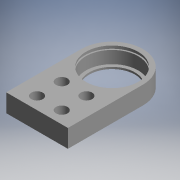
# Autodesk Inventor part: SBGSMA6006ZZ-40_h
Saved by Autodesk Inventor 2017.3 (Build 213256000, 256)
## iProperties
Part Number: SBGSMA6006ZZ-40_h
Material: Generic
Catalog Web Link: www.cadenas.de
Description: BGSMA, BGSMAB, SBGSMA_housing-Bearing with Housings - Front Installation Type
Vendor: MISUMI
Document SubType Name: Modeling
Designer: partserver
Manufacturer: MISUMI
Mass: 75.9528 g
Surface Area: 218.968 cm^2
Volume: 75.9528 cm^3
Density: 1 g/cm^3
Appearance: PSOLRGB-192-192-192
Category: PARTsolutions
Company: MISUMI
Title: SBGSMA6006ZZ-40
Author: Cadenas PARTsolutions
Comments: Bearing with Housings - Front Installation Type
PSOL_IDENT_0: {$CADENAS_DATA\23d-libs\misumi\metric\12_bearing_holders\bgsma\bgsma_housing.prj},219 {VTYP=3D},{NB=
PSOL_IDENT_1: SBGSMA6006ZZ-40_h},{LINA=SBGSMA6006ZZ-40},{NN=BGSMA, BGSMAB, SBGSMA_housing},{DATE=30.03.2018 01:48:
PSOL_IDENT_2: 31},{GEOMDATE=13.07.2015 10:26:00},{VERSION=},{LINEID=160},{WBVAR=MATB,STH,SEAL,HH,ALT1},{WBNUMERIC=
PSOL_IDENT_3: HH}  {NB=SBGSMA6006ZZ-40_h},{LINA=SBGSMA6006ZZ-40},{KT=DUMMY},{PN=SBGSMA6006ZZ-40},{TYPE=SBGSMA},{MA
PSOL_IDENT_4: TB=STS},{MATBALG= 'ST','Steel','STS','Stainless Steel' },{STH=},{STHALG= '','-' },{ARR=304 Stainless
PSOL_IDENT_5: Steel},{ARRALG=-S},{BN=6006},{SEAL=ZZ},{SEALALG= 'ZZ','ZZ(Double Shielded)','VV','VV(Non-contact Ru
PSOL_IDENT_6: bber Seal)','DD','DD(Contact Rubber Seal)' },{HH=40},{HHALG=40,45,55},{DD=30},{D=55},{DDHH=48},{B=13
PSOL_IDENT_7: },{H=111.5},{HH1=13},{L=65},{L1=26},{T=19},{DD1=12},{ALT1=},{ALT1ALG= '','Bearing and Retaining Ring
PSOL_IDENT_8: Assembled','NA','with NA (Bearing and Retaining Ring not Assembled)' },{ALT1PN=},{DD2=58.0},{TT=2.0
PSOL_IDENT_9: 0}
NB: SBGSMA6006ZZ-40_h
NN: BGSMA, BGSMAB, SBGSMA_housing
NT: Bearing with Housings - Front Installation Type
NBSYN: $PN._h
LINA: SBGSMA6006ZZ-40
CATALOG: Misumi
PN: SBGSMA6006ZZ-40
MATB: Stainless Steel
STH: -
ARR: 304 Stainless Steel
BN: 6006
SEAL: ZZ(Double Shielded)
HH: 40
DD: 30
D: 55
DDHH: 48
B: 13
H: 111.5
HH1: 13
L: 65
L1: 26
T: 19
DD1: 12
ALT1: Bearing and Retaining Ring Assembled
SUPPLIER: MISUMI
ARTICLENO: SBGSMA6006ZZ-40_h
BOMINFO: SBGSMA6006ZZ-40
CREATOR: CADENAS GmbH
Autodesk Inventor part; units mm, degrees
sketch "Sketch_7" plane through (0, 0, 0) normal (0, 0, 1) x (1, 0, 0)
  line L0 (-32.5, 79) -> (-32.5, 0)
  line L1 (-32.5, 0) -> (32.5, 0)
  line L2 (32.5, 0) -> (32.5, 79)
  arc A0 (32.5, 79) -> (-32.5, 79) centre (0, 79) ccw
  constraints: 6 end point, 2 point on circle, 1 centre point
extrude "Extrusion1" add sketch "Sketch_7" against normal blind 19
sketch "Sketch_8" plane through (0, 0, 0) normal (1, 0, 0) x (0, 0, -1)
  line L0 (19, 79) -> (2, 79)
  line L1 (2, 79) -> (2, 106.5)
  line L2 (2, 106.5) -> (15, 106.5)
  line L3 (15, 106.5) -> (15, 108)
  line L4 (15, 108) -> (17, 108)
  line L5 (17, 108) -> (17, 106.5)
  line L6 (17, 106.5) -> (19, 106.5)
  line L7 (19, 106.5) -> (19, 79)
  line L8 (19, 79) -> (2, 79)
  constraints: 18 end point
revolve "Revolution1" cut sketch "Sketch_8" angle 360 about axis through (0, 79, -19) along (0, 0, -1)
sketch "Sketch_1" plane through (0, 0, 0) normal (1, 0, 0) x (0, 0, -1)
  line L0 (19, 79) -> (0, 79)
  line L1 (0, 79) -> (0, 103)
  line L2 (0, 103) -> (19, 103)
  line L3 (19, 103) -> (19, 79)
  line L4 (19, 79) -> (0, 79)
  constraints: 10 end point
revolve "Revolution2" cut sketch "Sketch_1" angle 360 about axis through (0, 79, -19) along (0, 0, -1)
sketch "Sketch4" plane through (0, 0, -19) normal (0, 0, -1) x (-1, 0, 0)
  point P0 (13, 13)
hole "Hole1" at (-13, 13, -19) direction (0, 0, 1) diameter 12 depth 19
pattern_linear "Rectangular Pattern1" count 2 spacing 26 along (1, 0, 0) count 2 spacing 26 along (0, 1, 0) of "Hole1"
ref_plane "to_bearing_XY" through (0, 79, -8.5) normal (0, 0, 1) x (1, 0, 0)
ref_plane "to_bearing_YZ" through (0, 79, -8.5) normal (1, 0, 0) x (0, 1, 0)
ref_plane "to_bearing_ZX" through (0, 79, -8.5) normal (0, 1, 0) x (0, 0, 1)
ref_plane "to_retaining_ring_XY" through (0, 79, -17) normal (0, 0, -1) x (1, 0, 0)
ref_plane "to_retaining_ring_YZ" through (0, 79, -17) normal (1, 0, 0) x (0, -1, 0)
ref_plane "to_retaining_ring_ZX" through (0, 79, -17) normal (0, -1, 0) x (0, 0, -1)
body "Solid1"
